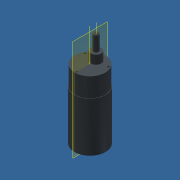
# Autodesk Inventor part: Conrad Motor
Saved by Autodesk Inventor 2014 SP2 (Build 180246200, 246)
## iProperties
Created: 2015-02-01
Part Number: Conrad Motor
Material: Eisen, grau
Document SubType Name: Modeling
Designer: 4ndreas
Density: 3.71179 g/cm^3
Appearance: Eisen - grau
Mass: 300 g
Surface Area: 117.609 cm^2
Volume: 80.8234 cm^3
Author: 4ndreas
Autodesk Inventor part; units mm, degrees
ref_plane "YZ Plane" through (0, 0, 0) normal (1, 0, 0) x (0, 1, 0)
ref_plane "XZ Plane" through (0, 0, 0) normal (0, 1, 0) x (-1, 0, 0)
ref_plane "XY Plane" through (0, 0, 0) normal (0, 0, 1) x (1, 0, 0)
sketch "Skizze1" plane through (0, 0, 0) normal (0, 0, 1) x (1, 0, 0)
  circle A0 centre (0, 0) radius 17.5
  dimension "d0" = 35
  constraints: 1 centre point, 1 coincident
  measures "d0" diameter of A0
extrude "Extrusion1" add sketch "Skizze1" against normal blind 22
sketch "Skizze2" plane through (0, 0, -22) normal (0, 0, -1) x (-1, 0, 0)
  circle A0 centre (0, 0) radius 17.5 projected
  circle A1 centre (0, 0) radius 18
  dimension "d3" = 36
  constraints: 1 centre point, 1 coincident
  measures "d3" diameter of A1
extrude "Extrusion2" add sketch "Skizze2" along normal blind 57.1 contours A0 | A1
sketch "Skizze3" plane through (0, 0, 0) normal (0, 0, 1) x (1, 0, 0)
  circle A0 centre (0, 0) radius 17.5 projected
  circle A1 centre (0, 7) radius 6
  line L0 (0, 0) -> (0, 7) construction
  dimension "d6" = 12
  dimension "d7" = 7
  constraints: 2 end point, 1 centre point, 1 vertical
  measures "d6" diameter of A1
  measures "d7" distance of L0.start L0.end
extrude "Extrusion3" add sketch "Skizze3" along normal blind 10 contours A1
sketch "Skizze4" plane through (0, 7, 10) normal (0, 0, 1) x (1, 0, 0)
  circle A0 centre (0, 0) radius 6 projected
  circle A1 centre (0, 0) radius 3
  point P0 (0, -7)
  dimension "d10" = 6
  constraints: 1 centre point, 1 coincident
  measures "d10" diameter of A1
extrude "Extrusion4" add sketch "Skizze4" along normal blind 17 contours A1
ref_plane "Arbeitsebene1" through (0, 7, 10) normal (1, 0, 0) x (0, 0, 1)
sketch "Skizze5" plane through (0, 0, 0) normal (0, 0, 1) x (1, 0, 0)
  circle A0 centre (0, 0) radius 17.5 projected
  circle A1 centre (0, 0) radius 15.5 construction
  line L0 (0, 0) -> (0, -17.5) construction
  line L1 (0, 0) -> (-15.1554, 8.75) construction
  line L2 (0, 0) -> (15.1554, 8.75) construction
  point P0 (-13.4234, 7.75)
  point P1 (13.4234, 7.75)
  point P2 (0, -15.5)
  dimension "d13" = 120
  dimension "d14" = 120
  dimension "d15" = 31
  constraints: 6 end point, 6 point on circle, 3 point on line, 1 centre point, 1 coincident, 1 vertical
  measures "d13" angle of L0 L1
  measures "d14" angle of L0 L2
  measures "d15" diameter of A1
hole "Bohrung1" at (-13.4234, 7.75, 0) at (13.4234, 7.75, 0) at (0, -15.5, 0) direction (0, 0, -1) diameter 2 depth 8
equation "\"d14\" = d13"
